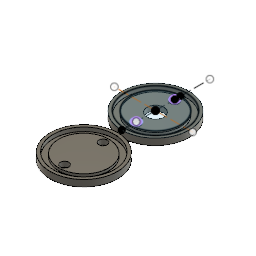
Pre+filter+housing (Autodesk Fusion 360 design; units mm, degrees)
Autodesk Fusion 360 part; units mm, degrees
sketch "Sketch5" plane through (0, 0, 0) normal (0, 1, 0) x (1, 0, 0)
  circle A0 centre (0, 0) radius 25.4
  dimension "d6" = 50.8
  constraint coincident A0.centre origin
  measures "d6" diameter of A0
extrude "Extrude1" add sketch "Sketch5" along normal blind 5 makes body 1
sketch "Sketch6" plane through (0, 5, 0) normal (0, 1, 0) x (-1, 0, 0)
  circle A0 centre (0, 0) radius 25.4
  circle A1 centre (0, 0) radius 18.8
  circle A2 centre (0, 0) radius 23.05
  line L0 (0, 0) -> (0, -41) construction
  line L1 (0, 0) -> (0, 25.4) construction
  circle A3 centre (0, -14.5) radius 3.15
  line L2 (-28, 0) -> (31, 0) construction
  circle A4 centre (0, 14.5) radius 3.15
  point P0 (0, -18.8)
  dimension "d9" = 37.6
  dimension "d10" = 46.1
  dimension "d21" = 6.3
  dimension "d22" = 4.3
  constraint coincident A0.centre A1.centre
  constraint vertical L0
  constraint coincident A0 L1.end
  constraint vertical L1
  constraint coincident L0 A3.centre
  constraint coincident A1 P0
  constraint coincident L0 P0
  constraint perpendicular L0 L2
  constraint symmetric A3 L2 A4
  measures "d9" diameter of A1
  measures "d10" diameter of A2
  measures "d21" diameter of A3
  measures "d22" distance of A3.centre P0
extrude "Extrude4" cut sketch "Sketch6" against normal blind 6 contours A3 | A4 bodies 1
extrude "Extrude2" cut sketch "Sketch6" against normal blind 3 contours A2 bodies 1
sketch "Sketch7" plane through (0, 5, 0) normal (0, 1, 0) x (-1, 0, 0)
  circle A0 centre (0, 0) radius 18.8
  circle A1 centre (0, -14.5) radius 3.15
  circle A2 centre (0, 14.5) radius 3.15
extrude "Extrude3" cut sketch "Sketch7" against normal blind 1 contours A0 | A1 | A2 bodies 1
copy_body "CopyPasteBodies1" bodies 1 makes body 2
move_body "Move1" bodies 2 to x (1, 0, 0) y (0, 1, 0) z (0, 0, 1) at (0, 0, 54)
hole "Hole3" at (0, 4, 0) direction (0, -1, 0) diameter 12.7 depth 5 tip angle 118 bodies 1
equation "d11 = 2 mm - 5 mm"
equation "d16 = 4 mm - 5 mm"
equation "d22 = 1.3 mm + 3 mm"
named bodies: "Upper", "Lower"
